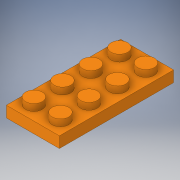
# Autodesk Inventor part: 2x4 orange pegged
Saved by Autodesk Inventor 2017 (Build 210142000, 142)
## iProperties
Created: 2018-05-15
Part Number: 2x4 orange pegged
Material: ABS Plastic
Document SubType Name: Modeling
Designer: 20000650
Density: 1.06 g/cm^3
Appearance: Orange
Author: 20000650
Autodesk Inventor part; units mm, degrees
ref_plane "YZ Plane" through (0, 0, 0) normal (1, 0, 0) x (0, 1, 0)
ref_plane "XZ Plane" through (0, 0, 0) normal (0, 1, 0) x (-1, 0, 0)
ref_plane "XY Plane" through (0, 0, 0) normal (0, 0, 1) x (1, 0, 0)
sketch "Sketch1" plane through (0, 0, 0) normal (0, 1, 0) x (-1, 0, 0)
  line L0 (0, 0) -> (0, -33.594)
  line L1 (0, -33.594) -> (15.5956, -33.594)
  line L2 (15.5956, -33.594) -> (15.5956, 0)
  line L3 (15.5956, 0) -> (0, 0)
  dimension "d0" = 33.594
  dimension "d1" = 15.5956
  dimension "d3" = 33.594
  constraints: 8 end point, 2 vertical, 1 perpendicular
  measures "d0" distance of L0.start L0.end
  measures "d1" distance of L0.end L1.end
  measures "d3" distance of L1.end L2.end
extrude "Extrusion1" add sketch "Sketch1" along normal blind 3.236
sketch "Sketch2" plane through (0, 3.236, 0) normal (0, 1, 0) x (1, 0, 0)
  line L0 (-15.5956, 33.594) -> (-15.5956, 0) projected
  line L1 (0, 0) -> (0, 33.594) projected
  line L2 (0, 33.594) -> (-15.5956, 33.594) projected
  line L3 (0, 33.594) -> (-15.5956, 33.594)
  line L4 (-15.5956, 0) -> (0, 0) projected
  circle A0 centre (-11.6967, 4.1993) radius 2.4498
  line L5 (-15.5956, 0) -> (0, 33.594)
  line L6 (-15.5956, 33.594) -> (0, 0)
  line L7 (-7.7978, 16.797) -> (-7.7978, 33.594)
  line L8 (-7.7978, 25.1955) -> (-7.7978, 16.797)
  line L9 (-7.7978, 0) -> (-7.7978, 16.797)
  line L10 (-7.7978, 8.3985) -> (-15.5956, 8.3985)
  line L11 (-15.5956, 8.3985) -> (-7.7978, 0)
  line L12 (-15.5956, 0) -> (-7.7978, 8.3985)
  dimension "d6" = 4.8997
  constraints: 18 end point, 5 midpoint, 3 collinear, 1 centre point, 1 perpendicular, 1 point on line
  measures "d6" diameter of A0
extrude "Extrusion2" add sketch "Sketch2" along normal blind 1.9837 contours L11 L5 A0 | A0 L5 L11 | L5 L11 L12 A0 | L12 L11 A0 | A0 L12 L11 L5 | A0 L11 L12
pattern_linear "Rectangular Pattern1" count 4 spacing 8.382 along (0, 0, -1) count 2 spacing 7.7978 along (1, 0, 0) of "Extrusion2"
shell "Shell1" thickness 1.4732 removed faces 1 at (-5.1985, 0, -22.396)
sketch "Sketch3" plane through (-14.1224, 1.7628, -1.4732) normal (0, -1, 0) x (1, 0, 0)
  circle A0 centre (10.2235, -2.7261) radius 2.4498 projected
  circle A1 centre (2.4257, -2.7261) radius 2.4498 projected
  circle A2 centre (10.2235, -27.8721) radius 0.9766 projected
  circle A3 centre (10.2235, -19.4901) radius 0.9766 projected
  circle A4 centre (10.2235, -11.1081) radius 0.9766 projected
  circle A5 centre (10.2235, -2.7261) radius 0.9766 projected
  circle A6 centre (2.4257, -27.8721) radius 0.9766 projected
  circle A7 centre (2.4257, -19.4901) radius 0.9766 projected
  circle A8 centre (2.4257, -11.1081) radius 0.9766 projected
  circle A9 centre (2.4257, -2.7261) radius 0.9766 projected
  line L0 (12.6492, 0) -> (12.6492, -30.6476) projected
  line L1 (0, 0) -> (12.6492, 0) projected
  line L2 (0, -30.6476) -> (0, 0) projected
  line L3 (12.6492, -30.6476) -> (0, -30.6476) projected
  circle A10 centre (2.4257, -11.1081) radius 2.4498 projected
  circle A11 centre (10.2235, -11.1081) radius 2.4498 projected
  circle A12 centre (10.2235, -19.4901) radius 2.4498 projected
  circle A13 centre (2.4257, -19.4901) radius 2.4498 projected
  circle A14 centre (2.4257, -27.8721) radius 2.4498 projected
  circle A15 centre (10.2235, -27.8721) radius 2.4498 projected
  circle A16 centre (6.3246, -6.9171) radius 3.2743
  circle A17 centre (6.3246, -15.3238) radius 3.2562
  circle A18 centre (6.3246, -23.6811) radius 3.2743
  circle A19 centre (6.3246, -6.9171) radius 2.4498
  circle A20 centre (6.3246, -15.3238) radius 2.4498
  circle A21 centre (6.3246, -23.6811) radius 2.4498
  point P0 (14.1224, 1.4732)
  dimension "d18" = 4.8997
  dimension "d19" = 4.8997
  dimension "d20" = 4.8997
  constraints: 6 centre point, 6 tangent, 3 coincident
  measures "d18" diameter of A19
  measures "d19" diameter of A20
  measures "d20" diameter of A21
extrude "Extrusion4" add sketch "Sketch3" along normal up to surface (1.7628 mm away) contours A16 | A17 | A18
body "Solid1"
